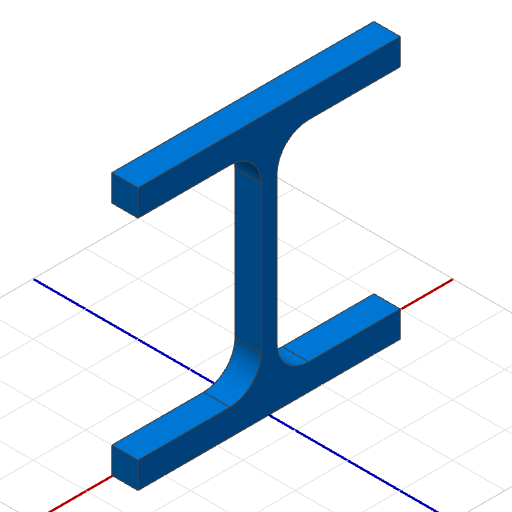
# Autodesk Inventor part: IPB
Saved by Autodesk Inventor 2023 (Build 270158000, 158)
## iProperties
Company: ТОВ "Свиспан Лімітед"
RuleStatus: InUse
Created: 2022-08-02
Part Number: IPB
Checked By: Жданюк Д.М.
Engr Approved By: Шевело В.М.
Material: Ст3сп ДСТУ 2651
Description: Деталь1
Document SubType Name: Modeling
Mfg Approved By: Янкевич О.Р.
Designer: Dima
Authority: Кудінкін Д.М.
Density: 7.85 g/cm^3
Appearance: С умеренной полировкой
Mass: 204.383 g
Surface Area: 108.812 cm^2
Volume: 26.0361 cm^3
AfterMaterialChange0: 2_Габарит деталі
BeforeDocSave0: 2_Габарит деталі
AfterAnyiPropertyChange0: 2_Габарит деталі
X_size: 100.0
Y_size: 100.0
Z_size: 10.0
Stren_steel: Ст3сп
Stan_steel: ДСТУ 2651
Author: Dima
Autodesk Inventor part; units mm, degrees
ref_plane "YZ Plane" through (0, 0, 0) normal (1, 0, 0) x (0, 1, 0)
ref_plane "XZ Plane" through (0, 0, 0) normal (0, 1, 0) x (-1, 0, 0)
ref_plane "XY Plane" through (0, 0, 0) normal (0, 0, 1) x (1, 0, 0)
sketch "Блок1" plane through (0, 0, 0) normal (0, 0, 1) x (1, 0, 0)
  line L0 (-15, -40) -> (-50, -40)
  line L1 (-50, -40) -> (-50, -50)
  arc A0 (-15, -40) -> (-3, -28) centre (-15, -28) ccw
  arc A1 (3, -28) -> (15, -40) centre (15, -28) ccw
  line L2 (50, -40) -> (15, -40)
  line L3 (-50, -50) -> (50, -50)
  line L4 (15, 40) -> (50, 40)
  line L5 (50, 50) -> (-50, 50)
  line L6 (50, 40) -> (50, 50)
  line L7 (3, -28) -> (3, 28)
  line L8 (-3, 28) -> (-3, -28)
  line L9 (-50, 40) -> (-15, 40)
  arc A2 (-3, 28) -> (-15, 40) centre (-15, 28) ccw
  arc A3 (15, 40) -> (3, 28) centre (15, 28) ccw
  line L10 (-50, 50) -> (-50, 40)
  line L11 (50, -50) -> (50, -40)
  line L12 (-3, 0) -> (3, 0) construction
  point P0 (0, 0)
  point P1 (3, 40)
  point P2 (-3, 40)
  point P3 (0, 0)
  dimension "d12" = 100
  dimension "d13" = 100
  dimension "d14" = 6
  dimension "d15" = 10
  dimension "d16" = 12
  measures "d12" distance between parallel lines of L3 L5
  measures "d13" distance of L1.end L11.start
  measures "d14" distance between parallel lines of L7 L8
  measures "d15" distance of L1.start L1.end
  measures "d16" radius of A2
sketch "Эскиз1" plane through (0, 0, 0) normal (0, 0, 1) x (1, 0, 0)
  line L0 (-3, 0) -> (3, 0) construction
  line L1 (-50, 40) -> (-15, 40)
  line L2 (-50, 50) -> (-50, 40)
  line L3 (50, 50) -> (-50, 50)
  line L4 (50, 40) -> (50, 50)
  line L5 (15, 40) -> (50, 40)
  line L6 (3, -28) -> (3, 28)
  line L7 (50, -40) -> (15, -40)
  line L8 (50, -50) -> (50, -40)
  line L9 (-50, -40) -> (-50, -50)
  line L10 (-15, -40) -> (-50, -40)
  line L11 (-3, 28) -> (-3, -28)
  arc A0 (-15, -40) -> (-3, -28) centre (-15, -28) ccw
  arc A1 (-3, 28) -> (-15, 40) centre (-15, 28) ccw
  arc A2 (15, 40) -> (3, 28) centre (15, 28) ccw
  arc A3 (3, -28) -> (15, -40) centre (15, -28) ccw
  line L12 (-50, -50) -> (50, -50)
  line L13 (0, 0) -> (0, 10) construction
  point P0 (-3, 40)
  point P1 (3, 40)
  dimension "d63" = 100
  dimension "d64" = 100
  dimension "d65" = 6
  dimension "d66" = 10
  dimension "d67" = 12
  dimension "d126" = 10
  dimension "d127" = 90
  constraints: 28 end point, 8 point on circle, 8 tangent, 6 collinear, 5 perpendicular, 4 centre point, 4 point on line, 3 equal radius, 3 midpoint, 1 vertical
  measures "d63" distance between parallel lines of L12 L3
  measures "d64" distance of L9.end L8.start
  measures "d65" distance between parallel lines of L6 L11
  measures "d66" distance of L9.start L9.end
  measures "d67" radius of A1
  measures "d126" distance of L13.start L13.end
  measures "d127" angle of L0 L13
extrude "Выдавливание5" add sketch "Эскиз1" along normal blind 10
equation "\"d12\" = ParH"
equation "\"d13\" = b"
equation "\"d14\" = t1"
equation "\"d15\" = t2"
equation "\"d16\" = R1"
equation "\"d63\" = ParH"
equation "\"d64\" = b"
equation "\"d65\" = t1"
equation "\"d66\" = t2"
equation "\"d67\" = R1"
equation "\"ParH\" = 100"
equation "\"b\" = 100"
equation "\"t1\" = 6"
equation "\"t2\" = 10"
equation "\"R1\" = 12"
equation "\"Height\" = 96"
equation "\"Thickness1\" = 5"
equation "\"Thickness2\" = 8"
